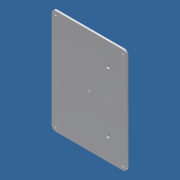
# Autodesk Inventor part: J001398
Saved by Autodesk Inventor 2012 SP2 (Build 160219200, 219)
## iProperties
Created: 2012-04-17
Part Number: J001398
Material: ALUMINUM, 6061-T651
Vendor: HHMI: JFRC - ID&F
Document SubType Name: Modeling
Designer: NEGRASHOVI
Density: 2.7 g/cm^3
Project: P-51601
Mass: 1537.22 g
Surface Area: 1891.35 cm^2
Volume: 569.342 cm^3
Description: CONTROLLER PLATE
RuleStatus: InUse
AfterDocSave0: file://Part Number Cleaner
LAB/DEPT: GONEN (LAB)
REQUESTING SCIENTIST: GONEN, TAMIR
SURFACE ROUGHNESS: 32 Ra
DESIGN DEPARTMENT: HHMI: JFRC - ID&F
SPECIAL FINISH: ANODIZE PER MIL-A-8625F, TYPE II, CLASS 2 (BLACK)
ALTERED ITEM PART NUMBER: N/A
ALTERED ITEM VENDOR: N/A
ALTERED ITEM DESCRIPTION: N/A
Author: NEGRASHOVI
Revision Number: -
Autodesk Inventor part; units mm, degrees
ref_plane "YZ Plane" through (0, 0, 0) normal (1, 0, 0) x (0, 1, 0)
ref_plane "XZ Plane" through (0, 0, 0) normal (0, 1, 0) x (-1, 0, 0)
ref_plane "XY Plane" through (0, 0, 0) normal (0, 0, 1) x (1, 0, 0)
sketch "Sketch1" plane through (0, 0, 0) normal (0, 0, 1) x (1, 0, 0)
  line L0 (-127, 177.8) -> (127, 177.8)
  line L1 (127, 177.8) -> (127, -177.8)
  line L2 (127, -177.8) -> (-127, -177.8)
  line L3 (-127, -177.8) -> (-127, 177.8)
  point P0 (0, 0)
  dimension "d0" = 254
  dimension "d1" = 127
  dimension "d2" = 355.6
  dimension "d3" = 177.8
  constraints: 8 end point, 2 parallel, 1 horizontal, 1 perpendicular
  measures "d0" distance of L0.start L0.end
  measures "d1" distance from line of L3 point (0, 0)
  measures "d2" distance of L0.end L1.end
  measures "d3" distance from line of point (0, 0) L0
extrude "Extrusion1" add sketch "Sketch1" along normal blind 6.35
sketch "Sketch2" plane through (0, 0, 6.35) normal (0, 0, 1) x (1, 0, 0)
  line L0 (-114.3, 165.1) -> (114.3, 165.1) construction
  line L1 (114.3, 165.1) -> (114.3, -165.1) construction
  line L2 (114.3, -165.1) -> (-114.3, -165.1) construction
  line L3 (-114.3, -165.1) -> (-114.3, 165.1) construction
  line L4 (-127, 177.8) -> (127, 177.8) construction
  line L5 (127, -177.8) -> (-127, -177.8) construction
  line L6 (-127, -177.8) -> (-127, 177.8) construction
  line L7 (127, 177.8) -> (127, -177.8) construction
  point P0 (0, 0)
  point P1 (0, 0)
  dimension "d6" = 12.7
  dimension "d7" = 12.7
  dimension "d8" = 12.7
  dimension "d9" = 12.7
  constraints: 8 end point, 5 coincident, 2 parallel, 1 horizontal, 1 perpendicular
  measures "d6" distance between parallel lines of L0 L4
  measures "d7" distance between parallel lines of L5 L2
  measures "d8" distance between parallel lines of L6 L3
  measures "d9" distance between parallel lines of L1 L7
hole "Hole1" at (-114.3, 165.1, 6.35) at (114.3, 165.1, 6.35) at (114.3, -165.1, 6.35) at (-114.3, -165.1, 6.35) at (0, 0, 6.35) direction (0, 0, -1) diameter 6.7564 end through all clearance for "Flat Head Machine Screw (82)" size "1/4" standard "Ansi Unified Screw Threads"
fillet "Fillet1" radius 12.7 4 edges at (127, -177.8, 3.175) (-127, -177.8, 3.175) (127, 177.8, 3.175) (-127, 177.8, 3.175)
sketch "Sketch9" plane through (127, -165.1, 0) normal (1, 0, 0) x (0, 0, -1)
  line L0 (-6.35, 330.2) -> (0, 330.2) projected
  line L1 (-6.35, 330.2) -> (-6.35, 0) projected
  line L2 (0, 0) -> (-6.35, 0) projected
  line L3 (0, 330.2) -> (0, 0) projected
  line L4 (-3.175, 330.2) -> (-3.175, 0) construction
  line L5 (0, 165.1) -> (-6.35, 165.1) construction
  point P0 (-3.175, 165.1)
  point P1 (-3.175, 311.15)
  point P2 (-3.175, 19.05)
  dimension "d68" = 146.05
  constraints: 4 end point, 4 midpoint, 2 point on line, 1 symmetric about line
  measures "d68" distance of point (-3.175, 311.15) point (-3.175, 165.1)
hole "Hole6" at (127, 0, 3.175) at (127, 146.05, 3.175) at (127, -146.05, 3.175) direction (-1, 0, 0) diameter 2.6416 depth 15.24 tip angle 118 thread size "6-32 UNC" class "2B" standard "ANSI Unified Screw Threads"
mirror "Mirror2" about plane through (0, 0, 0) normal (1, 0, 0) of "Hole6"
sketch "Sketch10" plane through (0, 0, 6.35) normal (0, 0, 1) x (1, 0, 0)
  line L0 (-177.8, 0) -> (177.8, 0) construction
  point P0 (0, 0)
  point P1 (86.36, 0)
  point P2 (38.1, 0)
  dimension "d76" = 48.26
  dimension "d85" = 38.1
  constraints: 2 point on line
  measures "d76" distance of point (86.36, 0) point (38.1, 0)
  measures "d85" distance of point (38.1, 0) point (0, 0)
hole "Hole7" at (86.36, 0, 6.35) at (38.1, 0, 6.35) direction (0, 0, -1) diameter 2.6416 end through all thread size "6-32 UNC" class "2B" standard "ANSI Unified Screw Threads"
sketch "Sketch11" plane through (0, 0, 6.35) normal (0, 0, 1) x (1, 0, 0)
  circle A0 centre (38.1, 0) radius 1.3208 projected
  circle A1 centre (86.36, 0) radius 1.3208 projected
  arc A2 (-114.3, 177.8) -> (-127, 165.1) centre (-114.3, 165.1) ccw projected
  line L0 (-127, -165.1) -> (-127, 165.1) projected
  arc A3 (-127, -165.1) -> (-114.3, -177.8) centre (-114.3, -165.1) ccw projected
  line L1 (114.3, -177.8) -> (-114.3, -177.8) projected
  arc A4 (114.3, -177.8) -> (127, -165.1) centre (114.3, -165.1) ccw projected
  line L2 (127, 165.1) -> (127, -165.1) projected
  arc A5 (127, 165.1) -> (114.3, 177.8) centre (114.3, 165.1) ccw projected
  line L3 (-114.3, 177.8) -> (114.3, 177.8) projected
  circle A6 centre (0, 0) radius 3.3782 projected
  circle A7 centre (-114.3, -165.1) radius 3.3782 projected
  circle A8 centre (114.3, -165.1) radius 3.3782 projected
  circle A9 centre (114.3, 165.1) radius 3.3782 projected
  circle A10 centre (-114.3, 165.1) radius 3.3782 projected
  line L4 (63.5, 177.8) -> (63.5, -177.8) construction
  line L5 (-127, 0) -> (127, 0) construction
  point P0 (63.5, 101.6)
  point P1 (63.5, -101.6)
  dimension "d86" = 63.5
  dimension "d87" = 101.6
  constraints: 4 end point, 4 point on line, 2 midpoint, 1 symmetric about line, 1 vertical
  measures "d86" distance from line of L4 point (0, 0)
  measures "d87" distance from line of point (63.5, 101.6) L5
hole "Hole8" at (63.5, 101.6, 6.35) at (63.5, -101.6, 6.35) direction (0, 0, -1) diameter 12.7 end through all
equation "\"d1\" = 0.5 * d0"
equation "\"d3\" = 0.5 * d2"
body "Solid1"
